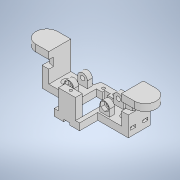
# Autodesk Inventor part: Основа рулевого механизма
Saved by Autodesk Inventor 2020 (Build 240168000, 168)
## iProperties
Created: 2021-03-14
Part Number: Основа рулевого механизма
Material: Типовые
Document SubType Name: Обычные детали
Designer: Антон
Density: 1 g/cm^3
Appearance: По умолчанию
Mass: 18.7306 g
Surface Area: 112.354 cm^2
Volume: 18.7306 cm^3
Sheet Metal Rule: По умолчанию
Author: Антон
Autodesk Inventor part; units mm, degrees
ref_plane "YZ Plane" through (0, 0, 0) normal (1, 0, 0) x (0, 1, 0)
ref_plane "XZ Plane" through (0, 0, 0) normal (0, 1, 0) x (-1, 0, 0)
sketch "Эскиз1" plane through (0, 0, 0) normal (0, 0, 1) x (1, 0, 0)
  line L0 (0, 0) -> (-17.5, 0)
  line L1 (-17.5, 0) -> (-17.5, 28.6)
  line L2 (-17.5, 28.6) -> (0, 28.6)
  line L3 (0, 28.6) -> (0, 0)
  line L4 (-17.5, 0) -> (-17.5, 5)
  line L5 (-17.5, 5) -> (-5, 5)
  line L6 (-5, 5) -> (-5, 23.6)
  line L7 (-5, 23.6) -> (-17.5, 23.6)
  line L8 (-17.5, 23.6) -> (-17.5, 5)
  line L9 (-5, 5) -> (0, 5)
  line L10 (-5, 5) -> (0, 5)
  line L11 (0, 5) -> (0, 3)
  line L12 (0, 3) -> (-5, 3)
  line L13 (-5, 3) -> (-5, 5)
  point P0 (0, 3)
  dimension "d8" = 17.5
  dimension "d9" = 28.6
  dimension "d10" = 5
  dimension "d11" = 12.5
  dimension "d12" = 18.6
  dimension "d353" = 2
  constraints: 28 end point, 6 parallel, 4 perpendicular, 4 point on line, 3 horizontal
  measures "d8" distance of L1.end L2.end
  measures "d9" distance of L0.end L1.end
  measures "d10" distance of L0.end L4.end
  measures "d11" distance of L7.end L6.end
  measures "d12" distance of L6.end L5.end
  measures "d353" distance of L10.end L11.end
extrude "Выдавливание1" add sketch "Эскиз1" along normal blind 16 contours L12 L13 L9 L3 | L9 L6 L7 L1 L2 L3
sketch "Эскиз4" plane through (-17.5, 23.6, 0) normal (0, -1, 0) x (1, 0, 0)
  line L0 (0, 0) -> (0, 16) projected
  line L1 (0, 8) -> (5, 8)
  circle A0 centre (5, 8) radius 4
  point P0 (17.5, 0)
  dimension "d31" = 5
  dimension "d32" = 8
  constraints: 2 end point, 1 centre point, 1 coincident, 1 horizontal, 1 midpoint
  measures "d31" distance of L1.start L1.end
  measures "d32" diameter of A0
extrude "Выдавливание2" cut sketch "Эскиз4" against normal blind 3
fillet "Сопряжение1" radius 8 2 edges at (-17.5, 26.1, 16) (-17.5, 26.1, 0)
sketch "Эскиз73" plane through (0, 28.6, 16) normal (0, 1, 0) x (1, 0, 0)
  line L0 (0, 16) -> (0, 0) projected
  circle A0 centre (-12.5, 8) radius 4 projected
  circle A1 centre (-12.5, 8) radius 4 projected
  line L1 (-21.3388, 11.8891) -> (-16.3891, 16.8388) construction
  line L2 (-16.3891, 16.8388) -> (-3.6612, 4.1109)
  line L3 (-3.6612, 4.1109) -> (-8.6109, -0.8388)
  line L4 (-8.6109, -0.8388) -> (-21.3388, 11.8891)
  line L5 (-21.3388, 11.8891) -> (-3.6612, 4.1109) construction
  line L6 (-16.3891, 16.8388) -> (-8.6109, -0.8388) construction
  line L7 (-12.5, 8) -> (-5, 8) construction
  line L8 (-5, 16) -> (-5, 0) construction
  circle A2 centre (9.7952, -0.8175) radius 3
  line L9 (-12.5, 8) -> (9.7952, -0.8175) construction
  line L10 (5.5525, -0.8175) -> (9.7952, 3.4251)
  line L11 (9.7952, 3.4251) -> (14.0378, -0.8175)
  line L12 (14.0378, -0.8175) -> (9.7952, -5.0602)
  line L13 (9.7952, -5.0602) -> (5.5525, -0.8175)
  line L14 (5.5525, -0.8175) -> (14.0378, -0.8175) construction
  line L15 (9.7952, 3.4251) -> (9.7952, -5.0602) construction
  line L16 (-8.6109, -0.8388) -> (9.7952, -5.0602)
  line L17 (-3.6612, 4.1109) -> (7.8426, 1.4726)
  line L18 (-12.5, 8) -> (3.0563, -7.5563) construction
  line L19 (3.0563, -7.5563) -> (9.7952, -0.8175) construction
  line L20 (-5, 16) -> (0, 16) projected
  line L21 (-5, 0) -> (0, 0) projected
  line L22 (-5, 16) -> (-5, 0) projected
  point P0 (9.7952, -0.8175)
  point P1 (0, 3.2712)
  point P2 (-8.6558, 9.1056)
  point P3 (-13.6056, 4.1558)
  dimension "d448" = 7
  dimension "d449" = 18
  dimension "d450" = 135
  dimension "d451" = 23.422
  dimension "d453" = 6
  dimension "d454" = 6
  dimension "d455" = 22
  constraints: 36 end point, 7 midpoint, 7 parallel, 3 perpendicular, 1 centre point, 1 coincident, 1 point on line, 1 tangent
  measures "d448" distance of L2.end L3.end
  measures "d449" distance of L1.end L2.end
  measures "d450" angle of L7 L2
  measures "d451" angle of L4 L9
  measures "d453" distance of L11.end L12.end
  measures "d454" distance of L10.end L11.end
  measures "d455" distance of L7.start L18.end
extrude "Выдавливание44" cut sketch "Эскиз73" against normal blind 6.1 from surface at -5 contours L17 L10 L13 L16 L3 L22 L21 L0 | L0 L21 L22 L3 L17 | L3 L22 L2 | L10 L11 A2 | L22 L3 L4 A0 L2 | A2 | A2 L13 L10 | L11 L12 A2 | A2 L12 L13
sketch "Эскиз70" plane through (-5, 3, 0) normal (0, -1, 0) x (1, 0, 0)
  line L0 (0, 0) -> (0, 16) construction
  line L1 (0, 8) -> (5, 8) construction
  line L2 (5, 0) -> (5, 16) construction
  line L3 (2.5, 3.5) -> (2.5, 12.5) construction
  point P0 (2.5, 8)
  dimension "d421" = 9
  constraints: 4 end point, 4 midpoint, 1 vertical
  measures "d421" distance of L3.start L3.end
hole "Отверстие22" at (-2.5, 3, 3.5) at (-2.5, 3, 12.5) direction (0, 1, 0) diameter 2.2 depth 6
sketch "Эскиз71" plane through (-5, 3, 0) normal (0, -1, 0) x (1, 0, 0)
  circle A0 centre (2.5, 3.5) radius 1.1 projected
  line L0 (3.597, 5.4) -> (4.6939, 3.5)
  line L1 (4.6939, 3.5) -> (3.597, 1.6)
  line L2 (3.597, 1.6) -> (1.403, 1.6)
  line L3 (1.403, 1.6) -> (0.3061, 3.5)
  line L4 (0.3061, 3.5) -> (1.403, 5.4)
  line L5 (1.403, 5.4) -> (3.597, 5.4)
  circle A1 centre (2.5, 12.5) radius 1.1 projected
  line L6 (3.597, 14.4) -> (4.6939, 12.5)
  line L7 (4.6939, 12.5) -> (3.597, 10.6)
  line L8 (3.597, 10.6) -> (1.403, 10.6)
  line L9 (1.403, 10.6) -> (0.3061, 12.5)
  line L10 (0.3061, 12.5) -> (1.403, 14.4)
  line L11 (1.403, 14.4) -> (3.597, 14.4)
  line L12 (0, 0) -> (0, 16) projected
  line L13 (0, 16) -> (5, 16) projected
  line L14 (0, 0) -> (5, 0) projected
  line L15 (1.403, 1.6) -> (0, 1.6)
  line L16 (0, 1.6) -> (0, 5.4)
  line L17 (0, 5.4) -> (1.403, 5.4)
  line L18 (1.403, 5.4) -> (1.403, 1.6)
  line L19 (1.403, 10.6) -> (0, 10.6)
  line L20 (0, 10.6) -> (0, 14.4)
  line L21 (0, 14.4) -> (1.403, 14.4)
  line L22 (1.403, 14.4) -> (1.403, 10.6)
  point P0 (0.4021, 3.3337)
  point P1 (0, 5.7805)
  point P2 (3.6, 3.5)
  point P3 (3.6, 3.5)
  point P4 (3.6, 12.5)
  point P5 (3.6, 12.5)
  point P6 (0, 1.6)
  point P7 (0, 10.6)
  dimension "d429" = 3.8
  constraints: 40 end point, 7 parallel, 3 point on line, 2 coincident, 2 horizontal, 2 perpendicular, 1 collinear, 26 other
  measures "d429" distance between parallel lines of L8 L11
extrude "Выдавливание42" cut sketch "Эскиз71" along normal blind 2 from surface at -6
sketch "Эскиз36" plane through (0, 3, 0) normal (0, -1, 0) x (1, 0, 0)
  line L0 (0, 0) -> (26.55, 0)
  line L1 (26.55, 0) -> (26.55, 16)
  line L2 (26.55, 16) -> (0, 16)
  line L3 (0, 16) -> (0, 0)
  dimension "d217" = 26.55
  constraints: 8 end point, 2 parallel, 1 coincident, 1 horizontal, 1 perpendicular
  measures "d217" distance of L2.end L1.end
extrude "Выдавливание23" add sketch "Эскиз36" against normal blind 5 from surface at 0
sketch "Эскиз66" plane through (0, 8, 0) normal (0, 1, 0) x (1, 0, 0)
  line L0 (0, 0) -> (0, -16) projected
  line L1 (0, -8) -> (5, -8)
  dimension "d396" = 5
  constraints: 2 end point, 1 horizontal, 1 midpoint
  measures "d396" distance of L1.start L1.end
hole "Отверстие20" at (5, 8, 8) direction (0, -1, 0) diameter 3.2 end through all countersink diameter 6 countersink angle 90
sketch "Эскиз67" plane through (0, 8, 0) normal (0, 1, 0) x (1, 0, 0)
  line L0 (10, -1.25) -> (17, -1.25)
  line L1 (17, -1.25) -> (17, -4.85)
  line L2 (17, -4.85) -> (10, -4.85)
  line L3 (10, -4.85) -> (10, -1.25)
  line L4 (10, -11.15) -> (17, -11.15)
  line L5 (17, -11.15) -> (17, -14.75)
  line L6 (17, -14.75) -> (10, -14.75)
  line L7 (10, -14.75) -> (10, -11.15)
  line L8 (13.5, -4.85) -> (13.5, -11.15) construction
  line L9 (26.55, -16) -> (26.55, 0) construction
  circle A0 centre (5, -8) radius 3 construction
  point P0 (0, 0)
  point P1 (13.5, -8)
  point P2 (26.55, -8)
  dimension "d404" = 7
  dimension "d405" = 3.6
  dimension "d406" = 6.3
  dimension "d407" = 2
  constraints: 18 end point, 4 midpoint, 4 parallel, 3 perpendicular, 2 equal length, 2 horizontal, 1 horizontal alignment
  measures "d404" distance of L0.start L0.end
  measures "d405" distance of L6.end L4.start
  measures "d406" distance between parallel lines of L4 L2
  measures "d407" distance edge to line of A0 L3
extrude "Выдавливание40" add sketch "Эскиз67" along normal blind 8.5
fillet "Сопряжение9" radius 3.5 4 edges at (10, 16.5, 3.05) (17, 16.5, 3.05) (10, 16.5, 12.95) (17, 16.5, 12.95)
sketch "Эскиз68" plane through (17, 8, 1.25) normal (0, 0, -1) x (-1, 0, 0)
  arc A0 (7, 5) -> (0, 5) centre (3.5, 5) ccw projected
  point P0 (17, -8)
hole "Отверстие21" at (13.5, 13, 1.25) direction (0, 0, 1) diameter 3.2 end through all countersink diameter 6 countersink angle 90
sketch "Эскиз69" plane through (10, 8, 14.75) normal (0, 0, 1) x (1, 0, 0)
  circle A0 centre (3.5, 5) radius 1.6 projected
  line L0 (3.5, 8.2332) -> (6.3, 6.6166)
  line L1 (6.3, 6.6166) -> (6.3, 3.3834)
  line L2 (6.3, 3.3834) -> (3.5, 1.7668)
  line L3 (3.5, 1.7668) -> (0.7, 3.3834)
  line L4 (0.7, 3.3834) -> (0.7, 6.6166)
  line L5 (0.7, 6.6166) -> (3.5, 8.2332)
  line L6 (0, 0) -> (0, 5) projected
  point P0 (3.5, 5)
  dimension "d462" = 5.6
  constraints: 12 end point, 1 coincident, 1 parallel, 13 other
  measures "d462" distance between parallel lines of L1 L4
extrude "Выдавливание41" cut sketch "Эскиз69" against normal blind 2.6
mirror "Зеркальное отражение6" about plane through (26.55, 3, 16) normal (1, 0, 0)
ref_plane "РабПлоскость6" through (26.55, 28.6, 16) normal (1, 0, 0) x (0, 0, -1)
sketch "Эскиз43" plane through (0, 0, 0) normal (0, 0, -1) x (-1, 0, 0)
  line L0 (-35.8, 8) -> (-17.3, 8)
  line L1 (-17.3, 8) -> (-17.3, 3)
  line L2 (-17.3, 3) -> (-35.8, 3)
  line L3 (-35.8, 3) -> (-35.8, 8)
  line L4 (-53.1, 8) -> (0, 8) projected
  line L5 (5, 3) -> (-58.1, 3) projected
  point P0 (-89.6, 0)
  point P1 (-26.55, 8)
  point P2 (0, 3)
  point P3 (-62.1, 3)
  point P4 (-53.1, 3)
  dimension "d260" = 18.5
  constraints: 8 end point, 2 collinear, 2 midpoint, 2 parallel, 1 horizontal, 1 perpendicular
  measures "d260" distance between parallel lines of L1 L3
extrude "Выдавливание27" add sketch "Эскиз43" along normal blind 4.45
sketch "Эскиз46" plane through (0, 0, 16) normal (0, 0, 1) x (1, 0, 0)
  line L0 (17.3, 8) -> (35.8, 8) projected
  line L1 (35.8, 3) -> (17.3, 3) projected
  line L2 (17.3, 3) -> (17.3, 8) projected
  line L3 (35.8, 8) -> (35.8, 3) projected
  point P0 (0, 0)
extrude "Выдавливание29" add sketch "Эскиз46" along normal blind 13.35
sketch "Эскиз48" plane through (0, 8, 16) normal (0, 1, 0) x (1, 0, 0)
  line L0 (20.3, -8.35) -> (32.8, -8.35)
  line L1 (32.8, -8.35) -> (32.8, 14.45)
  line L2 (32.8, 14.45) -> (20.3, 14.45)
  line L3 (20.3, 14.45) -> (20.3, -8.35)
  line L4 (35.8, -13.35) -> (17.3, -13.35) projected
  line L5 (17.3, -13.35) -> (35.8, -13.35) projected
  point P0 (0, 16)
  point P1 (19.525, -13.35)
  point P2 (0, 0)
  point P3 (26.55, -8.35)
  point P4 (26.55, -13.35)
  dimension "d280" = 12.5
  dimension "d281" = 22.8
  dimension "d458" = 5
  constraints: 8 end point, 2 midpoint, 2 parallel, 1 horizontal, 1 perpendicular, 1 vertical alignment
  measures "d280" distance of L1.end L2.end
  measures "d281" distance of L0.end L1.end
  measures "d458" distance between parallel lines of L4 L0
extrude "Выдавливание31" cut sketch "Эскиз48" against normal through all
sketch "Эскиз47" plane through (0, 8, 16) normal (0, 1, 0) x (1, 0, 0)
  line L0 (32.8, -13.35) -> (20.3, -13.35)
  line L1 (20.3, -13.35) -> (20.3, -8.35)
  line L2 (20.3, -8.35) -> (32.8, -8.35)
  line L3 (32.8, -8.35) -> (32.8, -13.35)
  line L4 (35.8, -13.35) -> (17.3, -13.35) projected
  line L5 (32.8, -8.35) -> (20.3, -8.35) projected
  line L6 (32.8, 14.45) -> (32.8, -8.35) projected
  point P0 (0, 16)
  point P1 (35.8, -12.35)
  point P2 (17.3, -12.35)
  point P3 (32.8, -7.35)
  point P4 (20.3, -7.35)
  point P5 (26.55, -8.35)
  point P6 (20.3, 15.45)
  point P7 (33.575, -13.35)
  point P8 (19.525, -13.35)
  point P9 (32.8, 19.45)
  constraints: 8 end point, 2 horizontal, 2 parallel, 1 midpoint, 1 perpendicular, 1 vertical, 4 other
extrude "Выдавливание30" add sketch "Эскиз47" along normal blind 14.6
sketch "Эскиз50" plane through (0, 22.6, 16) normal (0, 1, 0) x (1, 0, 0)
  line L0 (26.55, -8.35) -> (26.55, -10.425)
  line L1 (32.8, -8.35) -> (20.3, -8.35) projected
  point P0 (0, 16)
  point P1 (32.8, -7.35)
  point P2 (20.3, -7.35)
  dimension "d285" = 2.075
  constraints: 2 end point, 1 vertical, 2 other
  measures "d285" distance of L0.start L0.end
hole "Отверстие13" at (26.55, 22.6, 26.425) direction (0, -1, 0) diameter 2 depth 5 tip angle 118
sketch "Эскиз51" plane through (-11.5, 3, 9) normal (0, -1, 0) x (1, 0, 0)
  line L0 (44.3, -7.45) -> (31.8, -7.45) projected
  line L1 (44.3, -7.45) -> (42.05, -7.45)
  line L2 (31.8, -7.45) -> (34.05, -7.45)
  line L3 (42.05, -7.45) -> (42.05, -10.45)
  line L4 (34.05, -7.45) -> (34.05, -10.45)
  dimension "d459" = 3
  dimension "d461" = 8
  constraints: 8 end point, 2 equal length, 2 point on line, 2 vertical
  measures "d459" distance of L1.end L3.end
  measures "d461" distance between parallel lines of L4 L3
hole "Отверстие14" at (30.55, 3, -1.45) at (22.55, 3, -1.45) direction (0, 1, 0) diameter 2.2 end through all countersink diameter 4.2 countersink angle 90
sketch "Эскиз52" plane through (0, 8, 16) normal (0, 1, 0) x (1, 0, 0)
  line L0 (28.55, 14.45) -> (24.55, 14.45)
  line L1 (24.55, 14.45) -> (24.55, 16.45)
  line L2 (24.55, 16.45) -> (28.55, 16.45)
  line L3 (28.55, 16.45) -> (28.55, 14.45)
  line L4 (20.3, 14.45) -> (32.8, 14.45) projected
  point P0 (0, 16)
  point P1 (26.55, 14.45)
  point P2 (20.3, 15.45)
  point P3 (32.8, 15.45)
  dimension "d305" = 4
  dimension "d306" = 2
  constraints: 8 end point, 2 parallel, 1 horizontal, 1 midpoint, 1 perpendicular, 2 other
  measures "d305" distance of L1.end L2.end
  measures "d306" distance of L0.end L1.end
extrude "Выдавливание32" cut sketch "Эскиз52" against normal through all
sketch "Эскиз72" plane through (20.3, 3, 24.35) normal (0, 0, -1) x (-1, 0, 0)
  line L0 (-8.5, 1.5) -> (-4, 1.5)
  line L1 (-4, 1.5) -> (-4, 0)
  line L2 (-4, 0) -> (-8.5, 0)
  line L3 (-8.5, 0) -> (-8.5, 1.5)
  line L4 (0, 0) -> (-12.5, 0) projected
  point P0 (20.3, -3)
  point P1 (12.5, 0)
  point P2 (-6.25, 0)
  dimension "d432" = 1.5
  dimension "d433" = 4.5
  constraints: 8 end point, 2 midpoint, 2 parallel, 1 horizontal, 1 perpendicular
  measures "d432" distance of L0.end L1.end
  measures "d433" distance of L0.start L0.end
extrude "Выдавливание43" cut sketch "Эскиз72" against normal through all
fillet "Сопряжение11" radius 2.225 4 edges at (17.3, 5.5, 0) (17.3, 5.5, -4.45) (35.8, 5.5, -4.45) (35.8, 5.5, 0)
equation "\"d10\" = -0.5 * d12 + 0.5 * d9"
